side_short_with_ports_v23 (Autodesk Fusion 360 design; units mm, degrees)
Autodesk Fusion 360 part; units mm, degrees
note: some values were not read from the file. Set by a fixed rule: which sketch regions a step uses.
sketch "Sketch1" plane through (0, 0, 0) normal (1, 0, 0) x (0, 0, -1)
  line L0 (0, 0) -> (226.726, 0)
  line L1 (226.726, 0) -> (226.726, 70.4)
  line L2 (226.726, 70.4) -> (0, 70.4)
  line L3 (0, 70.4) -> (0, 0)
  line L4 (5.4, 0) -> (25.3, 0)
  line L5 (25.3, 0) -> (25.3, 32.4)
  line L6 (25.3, 32.4) -> (5.4, 32.4)
  line L7 (5.4, 32.4) -> (5.4, 0)
  line L8 (103.413, 0) -> (123.313, 0)
  line L9 (123.313, 0) -> (123.313, 32.4)
  line L10 (123.313, 32.4) -> (103.413, 32.4)
  line L11 (103.413, 32.4) -> (103.413, 0)
  line L12 (221.326, 0) -> (201.426, 0)
  line L13 (201.426, 0) -> (201.426, 32.4)
  line L14 (201.426, 32.4) -> (221.326, 32.4)
  line L15 (221.326, 32.4) -> (221.326, 0)
  dimension "d1" = 226.726
  dimension "d2" = 70.4
  dimension "d3" = 19.9
  dimension "d4" = 19.9
  dimension "d5" = 19.9
  dimension "d6" = 5.4
  dimension "d7" = 5.4
  dimension "d8" = 32.4
  dimension "d9" = 32.4
  dimension "d10" = 32.4
  dimension "d11" = 103.413
  constraint horizontal L0
  constraint vertical L1
  constraint horizontal L2
  constraint vertical L3
  constraint coincident L0.start L3.end
  constraint horizontal L4
  constraint vertical L5
  constraint horizontal L6
  constraint vertical L7
  constraint coincident L0 L4.start
  constraint horizontal L8
  constraint vertical L9
  constraint horizontal L10
  constraint vertical L11
  constraint coincident L0 L8.start
  constraint horizontal L12
  constraint vertical L13
  constraint horizontal L14
  constraint vertical L15
  constraint coincident L0 L12.start
  measures "d1" distance of L0.start L0.end
  measures "d2" distance of L0.start L2.end
  measures "d3" distance of L5.end L6.end
  measures "d4" distance of L9.end L10.end
  measures "d5" distance of L13.end L14.end
  measures "d6" distance of L3 L7
  measures "d7" distance of L1 L15
  measures "d8" distance of L4.start L6.end
  measures "d9" distance of L8.start L10.end
  measures "d10" distance of L12.end L13.end
  measures "d11" distance of L1 L9
extrude "Extrude1" add sketch "Sketch1" along normal blind 5.4 contours L0 L1 L2 L3 L5 L6 L7 L9 L10 L11 L13 L14 L15
sketch "Sketch2" plane through (5.4, 0, 0) normal (1, 0, 0) x (0, 0, -1)
  line L0 (123.313, 0) -> (201.426, 0)
  line L1 (201.426, 0) -> (201.426, 32.4)
  line L2 (201.426, 32.4) -> (221.326, 32.4)
  line L3 (221.326, 32.4) -> (221.326, 0)
  line L4 (221.326, 0) -> (226.726, 0)
  line L5 (226.726, 0) -> (226.726, 70.4)
  line L6 (226.726, 70.4) -> (0, 70.4)
  line L7 (0, 70.4) -> (0, 0)
  line L8 (0, 0) -> (5.4, 0)
  line L9 (5.4, 0) -> (5.4, 32.4)
  line L10 (5.4, 32.4) -> (25.3, 32.4)
  line L11 (25.3, 32.4) -> (25.3, 0)
  line L12 (25.3, 0) -> (103.413, 0)
  line L13 (103.413, 0) -> (103.413, 32.4)
  line L14 (103.413, 32.4) -> (123.313, 32.4)
  line L15 (123.313, 32.4) -> (123.313, 0)
  line L16 (27.4, 32.4) -> (102.3, 32.4) construction
  line L17 (102.3, 32.4) -> (102.3, 0) construction
  line L18 (102.3, 0) -> (27.4, 0) construction
  line L19 (27.4, 0) -> (27.4, 32.4) construction
  line L20 (30.4, 29.3) -> (42.6, 29.3)
  line L21 (42.6, 29.3) -> (42.6, 9.1)
  line L22 (42.6, 9.1) -> (30.4, 9.1)
  line L23 (30.4, 9.1) -> (30.4, 29.3)
  circle A0 centre (72.45, 26.4) radius 4.85
  line L24 (56.7, 20.75) -> (88.2, 20.75)
  line L25 (88.2, 20.75) -> (88.2, 6)
  line L26 (88.2, 6) -> (56.7, 6)
  line L27 (56.7, 6) -> (56.7, 20.75)
  line L28 (72.45, 6) -> (72.45, 20.75) construction
  line L29 (72.45, 31.25) -> (72.45, 21.55) construction
  line L30 (79.45, 20.4) -> (65.45, 20.4) construction
  line L31 (65.45, 20.4) -> (65.45, 32.4) construction
  line L32 (65.45, 32.4) -> (79.45, 32.4) construction
  line L33 (79.45, 32.4) -> (79.45, 20.4) construction
  line L34 (79.45, 20.4) -> (65.45, 32.4) construction
  line L35 (65.45, 20.4) -> (79.45, 32.4) construction
  line L36 (25.3, 6) -> (103.413, 6) construction
  point P0 (72.45, 26.4)
  dimension "d15" = 77
  dimension "d16" = 12.2
  dimension "d17" = 20.2
  dimension "d26" = 9.7
  dimension "d27" = 31.5
  dimension "d28" = 14.75
  dimension "d34" = 3
  dimension "d35" = 3.1
  dimension "d36" = 32.4
  dimension "d37" = 14
  dimension "d38" = 12
  dimension "d39" = 6
  dimension "d42" = 59.7
  dimension "d43" = 29.85
  dimension "d49" = 22
  constraint horizontal L16
  constraint vertical L17
  constraint horizontal L18
  constraint vertical L19
  constraint coincident L11.end L18
  constraint collinear L10 L16
  constraint horizontal L20
  constraint vertical L21
  constraint horizontal L22
  constraint vertical L23
  constraint horizontal L24
  constraint vertical L25
  constraint horizontal L26
  constraint vertical L27
  constraint midpoint L26 L28.start
  constraint midpoint L24 L28.end
  constraint coincident A0 L29.start
  constraint perpendicular L12 L29
  constraint collinear L28 L29
  constraint horizontal L30
  constraint perpendicular L30 L31
  constraint parallel L30 L32
  constraint parallel L31 L33
  constraint coincident L34 P0
  constraint coincident L35 P0
  constraint coincident P0 A0.centre
  constraint coincident P0 L29
  constraint coincident A0 L29.end
  constraint coincident L11 L36.start
  constraint perpendicular L11 L36
  constraint coincident L13 L36.end
  constraint collinear L16 L32
  constraint collinear L26 L36
  measures "d15" distance of L11 L17
  measures "d16" distance of L20.start L20.end
  measures "d17" distance of L20.start L22.end
  measures "d26" diameter of A0
  measures "d27" distance of L24.start L24.end
  measures "d28" distance of L24.start L26.end
  measures "d34" distance of L19 L23
  measures "d35" distance of L16 L20
  measures "d36" distance of L8.end L9.end
  measures "d37" distance of L31.end L32.end
  measures "d38" distance of L30.end L31.end
  measures "d39" distance of L12 L36
  measures "d42" distance of L17 L21
  measures "d43" distance of L21 P0
  measures "d49" distance of L9 L19
sketch "Sketch3" plane through (5.4, 0, 0) normal (1, 0, 0) x (0, 0, -1)
  line L0 (73.363, 22.4) -> (153.363, 22.4)
  arc A0 (153.363, 22.4) -> (153.363, 32.4) centre (153.363, 27.4) ccw
  line L1 (153.363, 32.4) -> (73.363, 32.4)
  arc A1 (73.363, 32.4) -> (73.363, 22.4) centre (73.363, 27.4) ccw
  line L2 (73.363, 27.4) -> (153.363, 27.4) construction
  line L3 (226.726, 70.4) -> (0, 70.4)
  line L4 (0, 70.4) -> (0, 0)
  line L5 (123.313, 0) -> (201.426, 0)
  line L6 (103.413, 32.4) -> (103.413, 22.4)
  line L7 (25.3, 32.4) -> (25.3, 0)
  line L8 (103.413, 32.4) -> (123.313, 32.4)
  line L9 (103.413, 0) -> (103.413, 32.4)
  point P0 (113.363, 27.4)
  dimension "d18" = 5
  dimension "d19" = 80
  dimension "d20" = 226.726
  dimension "d21" = 113.363
  constraint tangent L0 A0
  constraint tangent A0 L1
  constraint parallel L0 L1
  constraint tangent L1 A1
  constraint tangent L0 A1
  constraint horizontal L2
  constraint midpoint L2 P0
  constraint coincident L1 L6.start
  constraint coincident L0 L6.end
  constraint perpendicular L0 L6
  constraint collinear L1 L8
  constraint collinear L6 L9
  measures "d18" radius of A0
  measures "d19" distance of A1.centre A0.centre
  measures "d20" distance of L3.start L3.end
  measures "d21" distance of P0 L4
extrude "Extrude2" cut sketch "Sketch3" against normal blind 55 contours L0 A0 L1 L6 L8 L9
extrude "Extrude3" cut sketch "Sketch2" against normal blind 10 contours L20 L21 L22 L23 | A0 | L24 L25 L26 L27
sketch "exoprt" plane through (5.4, 0, 0) normal (1, 0, 0) x (0, 0, -1)
  line L0 (42.6, 29.3) -> (42.6, 9.1)
  line L1 (42.6, 9.1) -> (30.4, 9.1)
  line L2 (30.4, 9.1) -> (30.4, 29.3)
  line L3 (30.4, 29.3) -> (42.6, 29.3)
  line L4 (88.2, 20.75) -> (88.2, 6)
  line L5 (88.2, 6) -> (56.7, 6)
  line L6 (56.7, 6) -> (56.7, 20.75)
  line L7 (56.7, 20.75) -> (88.2, 20.75)
  circle A0 centre (72.45, 26.4) radius 4.85
  line L8 (153.363, 22.4) -> (123.313, 22.4)
  line L9 (123.313, 22.4) -> (123.313, 0)
  line L10 (123.313, 0) -> (201.426, 0)
  line L11 (201.426, 0) -> (201.426, 32.4)
  line L12 (201.426, 32.4) -> (221.326, 32.4)
  line L13 (221.326, 32.4) -> (221.326, 0)
  line L14 (221.326, 0) -> (226.726, 0)
  line L15 (226.726, 0) -> (226.726, 70.4)
  line L16 (226.726, 70.4) -> (0, 70.4)
  line L17 (0, 70.4) -> (0, 0)
  line L18 (0, 0) -> (5.4, 0)
  line L19 (5.4, 0) -> (5.4, 32.4)
  line L20 (5.4, 32.4) -> (25.3, 32.4)
  line L21 (25.3, 32.4) -> (25.3, 0)
  line L22 (25.3, 0) -> (103.413, 0)
  line L23 (103.413, 0) -> (103.413, 32.4)
  line L24 (103.413, 32.4) -> (153.363, 32.4)
  arc A1 (153.363, 22.4) -> (153.363, 32.4) centre (153.363, 27.4) ccw
equation "d2 = d8 + 38 mm"
equation "d4 = d3"
equation "d5 = d4"
equation "d7 = d6"
equation "d8 = 6 * 5.4 mm"
equation "d9 = d8"
equation "d10 = d9"
equation "d11 = ( d1 - d4 ) / 2"
equation "d21 = d20 / 2"
equation "d35 = ( d36 - d39 - d17 ) / 2"
equation "d43 = d42 / 2"
